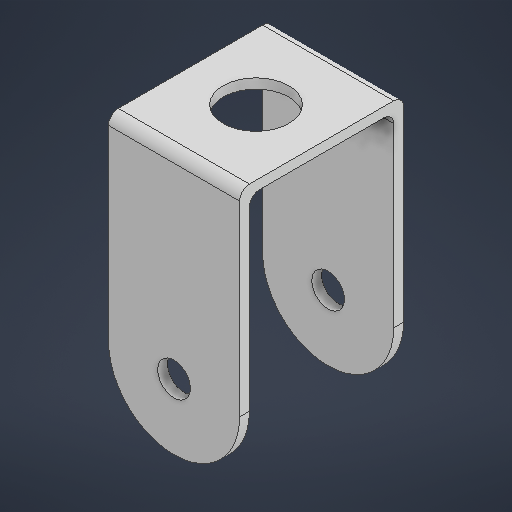
# Autodesk Inventor part: Peça2
Saved by Autodesk Inventor 2027 (Build 310192060, 192F)
## iProperties
Created: 2026-08-06
Part Number: Peça2
Material: Genérico
Document SubType Name: Modeling
Designer: labsfiap
Density: 1 g/cm^3
Appearance: Padrão
Author: labsfiap
Autodesk Inventor part; units mm, degrees
ref_plane "YZ Plane" through (0, 0, 0) normal (1, 0, 0) x (0, 1, 0)
ref_plane "XZ Plane" through (0, 0, 0) normal (0, 1, 0) x (-1, 0, 0)
ref_plane "XY Plane" through (0, 0, 0) normal (0, 0, 1) x (1, 0, 0)
sketch "Esboço1" plane through (0, 0, 0) normal (1, 0, 0) x (0, 1, 0)
  line L0 (0, 0) -> (16.1325, 0)
  line L1 (80, -25) -> (0, -25)
  line L2 (0, -25) -> (0, -22)
  line L3 (80, -25) -> (80, 25)
  line L4 (80, 25) -> (0, 25)
  line L5 (0, 25) -> (0, 22)
  line L6 (0, 22) -> (77, 22)
  line L7 (77, 22) -> (77, -22)
  line L8 (77, -22) -> (0, -22)
  constraints: 18 end point, 4 perpendicular, 2 horizontal, 1 parallel, 1 vertical
extrude "Extrusão1" add sketch "Esboço1" along normal blind 40
fillet "Arredondamento1" radius 20 4 edges at (0, 0, -23.5) (40, 0, -23.5) (0, 0, 23.5) (40, 0, 23.5)
fillet "Arredondamento2" radius 3 4 edges at (20, 80, -25) (20, 80, 25) (20, 77, -22) (20, 77, 22)
sketch "Esboço2" plane through (20, 20, -25) normal (0, 0, -1) x (-1, 0, 0)
  line L0 (-20, 60) -> (20, 60) projected
  line L1 (0, 60) -> (0, 0)
  circle A0 centre (0, 0) radius 5
  point P0 (20, -20)
  dimension "d17" = 60
  dimension "d18" = 10
  constraints: 2 end point, 1 centre point, 1 coincident, 1 midpoint, 1 vertical
  measures "d17" distance of L1.start L1.end
  measures "d18" diameter of A0
extrude "Extrusão2" cut sketch "Esboço2" against normal through all
sketch "Esboço3" plane through (0, 80, 22) normal (0, 1, 0) x (1, 0, 0)
  line L0 (40, 44) -> (40, 0) projected
  line L1 (40, 22) -> (0, 22)
  circle A0 centre (20, 22) radius 10
  dimension "d21" = 20
  constraints: 2 end point, 2 midpoint, 1 centre point, 1 horizontal
  measures "d21" diameter of A0
extrude "Extrusão3" cut sketch "Esboço3" against normal blind 10
